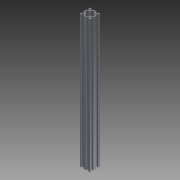
# Autodesk Inventor part: HFS5-4040-530
Saved by Autodesk Inventor 2015 (Build 190159000, 159)
## iProperties
Category: PARTsolutions
Company: MISUMI
Created: 2014-03-18
Part Number: HFS5-4040-530
Catalog Web Link: www.cadenas.de
Description: NFS5-4040, NFSB5-4040, HFS5-4040, HFSB5-4040, CAF5-4040, NFSF5-4040, HFSF5-4040,  HFST5-4040-HFS5 Series Aluminum Extrusions 40mm Square -2 Slots-
Vendor: MISUMI
Document SubType Name: Modeling
Designer: PARTuser1
Manufacturer: MISUMI
Density: 1 g/cm^3
Material: Generic
Appearance: RGB(175.94999939203154,175.94999939203154,175.94999939203154)
PSOL_IDENT_0: {\\10.0.0.236\data_v8\23d-libs\misumi\metric\38_al_extrusions_blackets\5\hfs5_4040.prj},542 {VTYP=3D
PSOL_IDENT_1: },{NB=HFS5-4040-530},{LINA=HFS5-4040-530},{NN=NFS5-4040, NFSB5-4040, HFS5-4040, HFSB5-4040, CAF5-404
PSOL_IDENT_2: 0, NFSF5-4040, HFSF5-4040,  HFST5-4040},{DATE=26.12.2013 07:39:21},{GEOMDATE=11.12.2013 08:22:00},{V
PSOL_IDENT_3: ERSION=},{LINEID=130},{LINESUBID=-1},{WBVAR=L,ALT1,ALT2,ALT4,ALT5,CP5,DL5,DR5,ALT6,HP6,NHL6,DL6,NHR6
PSOL_IDENT_4: ,DR6,ALT7,ALT8,ALT9,ALT10,ALT11,NH9,AH,BH,CH,DH,EH,NH10,AV,BV,CV,DV,EV,NH11,AP,BP,CP,DP,EP,ALT12,ALT
PSOL_IDENT_5: 13,Z,NH12,XA,XB,XC,XD,XE,NH13,YA,YB,YC,YD,YE,ALT16,HP16,DL16,DR16,ALT17,HQ17,JLP,ALT18,HQ18,KLP,ALT2
PSOL_IDENT_6: 0,ALT21,CHARSELECT1,CHARSELECT2}  {NB=HFS5-4040-530},{LINA=HFS5-4040-530},{KT=DUMMY},{PN=HFS5-4040-5
PSOL_IDENT_7: 30},{TPS=HFS5-4040},{MAT=A6N01SS-T5 Aluminum Alloy},{ST=Clear Anodize},{FRMW=40},{FRMH=40},{FRD=4.2}
PSOL_IDENT_8: ,{L=530.0},{MASS=1.28},{SA=472},{LX=8.89x10^4},{LY=8.89x10^4},{ALT1=},{M1=0},{DPL1=0},{DPR1=0},{ALT1
PSOL_IDENT_9: PN=},{ALT2=},{ALT2ALG= '','w/o End Tapping (Heli-Coil Insert)','LHP','with LHP (Tapping on the Left
PSOL_IDENT_10: (Heli-Coil Insert))','RHP','with RHP (Tapping on the Right (Heli-Coil Insert))','HPW','with HPW (Tap
PSOL_IDENT_11: ping on Both Ends (Heli-Coil Insert))' },{M2=0},{DP2=0},{ALT2PN=},{ALT4=},{ALT4ALG= '', 'w/o SC (Hig
PSOL_IDENT_12: h Precision Cut)', 'SC', 'with SC (High Precision Cut)' },{ALT4PN=},{ALT5=},{ALT5ALG= '','w/o 45 Deg
PSOL_IDENT_13: ree Cut','1','with 45 Degree Cut' },{CP5=},{CP5ALG= '','N/A' },{DL5=},{DL5ALG= '','N/A' },{DR5=},{DR
PSOL_IDENT_14: 5ALG= '','N/A' },{FRMALT5=0},{ALT5PN=},{ALT6=},{ALT6ALG= '','w/o Fastening Location Wrench Access Ho
PSOL_IDENT_15: le Alterations','1','with Fastening Location Wrench Access Hole Alterations' },{DD6=0.00},{HP6=},{HP
PSOL_IDENT_16: 6ALG= '','N/A' },{NHL6=},{NHL6ALG= '','N/A' },{DL6=},{DL6ALG= '','N/A' },{NHR6=},{NHR6ALG= '','N/A'
PSOL_IDENT_17: },{DR6=},{DR6ALG= '','N/A' },{HL6=0},{HR6=0},{J6=0},{K6=0},{ALT7=},{ALT7ALG= '','N/A' },{ALT8=},{ALT
PSOL_IDENT_18: 8ALG= '','N/A' },{ALT678PN=},{ALT9=},{ALT9ALG= '','w/o Location Specified Wrench Access Hole Alterat
PSOL_IDENT_19: ons (Horizontal)','1','with Location Specified Wrench Access Hole Alteratons (Horizontal)' },{ALT10=
PSOL_IDENT_20: },{ALT10ALG= '','w/o Location Specified Wrench Access Hole Alteratons (Vertical)','1','with Location
PSOL_IDENT_21: Specified Wrench Access Hole Alteratons (Vertical)' },{ALT11=},{ALT11ALG= '','w/o Location Specifie
PSOL_IDENT_22: d Wrench Access Hole Alteratons (Crisscross)','1','with Location Specified Wrench Access Hole Altera
PSOL_IDENT_23: tons (Crisscross)' },{DD9=0.00},{NH9=0},{NH9MAX=5},{NH9ALG=[0]},{AH=0.0},{AHMIN=7},{AHMAX=525},{AHAL
PSOL_IDENT_24: G=[0]},{BH=0.0},{BHMIN=2},{BHMAX=527},{BHALG=[0]},{CH=0.0},{CHMIN=2},{CHMAX=529},{CHALG=[0]},{DH=0.0
PSOL_IDENT_25: },{DHMIN=2},{DHMAX=531},{DHALG=[0]},{EH=0.0},{EHMIN=2},{EHMAX=523},{EHALG=[0]},{NH10=0},{NH10MAX=5},
PSOL_IDENT_26: {NH10ALG=[0]},{AV=0.0},{AVMIN=7},{AVMAX=525},{AVALG=[0]},{BV=0.0},{BVMIN=2},{BVMAX=527},{BVALG=[0]},
PSOL_IDENT_27: {CV=0.0},{CVMIN=2},{CVMAX=529},{CVALG=[0]},{DV=0.0},{DVMIN=2},{DVMAX=531},{DVALG=[0]},{EV=0.0},{EVMI
PSOL_IDENT_28: N=2},{EVMAX=523},{EVALG=[0]},{NH11=0},{NH11MAX=5},{NH11ALG=[0]},{AP=0.0},{APMIN=7},{APMAX=525},{APAL
PSOL_IDENT_29: G=[0]},{BP=0.0},{BPMIN=2},{BPMAX=527},{BPALG=[0]},{CP=0.0},{CPMIN=2},{CPMAX=529},{CPALG=[0]},{DP=0.0
PSOL_IDENT_30: },{DPMIN=2},{DPMAX=531},{DPALG=[0]},{EP=0.0},{EPMIN=2},{EPMAX=523},{EPALG=[0]},{ALT9PN=},{ALT10PN=},
PSOL_IDENT_31: {ALT11PN=},{ALT91011PN=},{ALT12=},{ALT12ALG= '','w/o Counterbore Hole in Specified Position (Vertica
PSOL_IDENT_32: l)','1','with Counterbore Hole in Specified Position (Vertical)' },{ALT13=},{ALT13ALG= '','w/o Count
PSOL_IDENT_33: erbore Hole in Specified Position (Horizontal)','1','with Counterbore Hole in Specified Position (Ho
PSOL_IDENT_34: rizontal)' },{Z=},{ZALG= '','N/A' },{DD12=0.0},{DD112=0.0},{NH12=0},{NH12MAX=5},{NH12ALG=[0]},{XA=0.
PSOL_IDENT_35: 0},{XAMIN=7},{XAMAX=525},{XAALG=[0]},{XB=0.0},{XBMIN=2},{XBMAX=527},{XBALG=[0]},{XC=0.0},{XCMIN=2},{
PSOL_IDENT_36: XCMAX=529},{XCALG=[0]},{XD=0.0},{XDMIN=2},{XDMAX=531},{XDALG=[0]},{XE=0.0},{XEMIN=2},{XEMAX=523},{XE
PSOL_IDENT_37: ALG=[0]},{NH13=0},{NH13MAX=5},{NH13ALG=[0]},{YA=0.0},{YAMIN=7},{YAMAX=525},{YAALG=[0]},{YB=0.0},{YBM
PSOL_IDENT_38: IN=2},{YBMAX=527},{YBALG=[0]},{YC=0.0},{YCMIN=2},{YCMAX=529},{YCALG=[0]},{YD=0.0},{YDMIN=2},{YDMAX=5
PSOL_IDENT_39: 31},{YDALG=[0]},{YE=0.0},{YEMIN=2},{YEMAX=523},{YEALG=[0]},{ALT12PN=},{ALT13PN=},{ALT1213PN=},{ALT16
PSOL_IDENT_40: =},{ALT16ALG= '','w/o M Type Hole Alteration','1','with M Type Hole Alteration' },{HP16=},{HP16ALG=
PSOL_IDENT_41: '','N/A' },{DL16=},{DL16ALG= '','N/A' },{DR16=},{DR16ALG= '','N/A' },{H116=0},{D16=0.0},{ALT16PN=},{
PSOL_IDENT_42: ALT17=},{ALT17ALG= '','w/o L Type Hole Alteration (Top)','1','with L Type Hole Alteration (Top)' },{
PSOL_IDENT_43: HQ17=0},{HQ17ALG=0},{JLP=0},{JLPMIN=4.9},{JLPMAX=0},{JLPALG=[0]},{L17=0},{D17=0.0},{ALT17PN=},{ALT18
PSOL_IDENT_44: =},{ALT18ALG= '','w/o L Type Hole Alteration (Bottom)','1','with L Type Hole Alteration (Bottom)' },
PSOL_IDENT_45: {HQ18=0},{HQ18ALG=0},{KLP=0},{KLPMIN=4.9},{KLPMAX=0},{KLPALG=[0]},{L18=0},{D18=0.0},{ALT18PN=},{ALT2
PSOL_IDENT_46: 0=},{ALT20PN=},{ALT21=},{CHARSELECT1=},{CS1=},{CHARSELECT2=},{CS2=},{ALT21PN=},{ERRORALT01=OK},{ERRO
PSOL_IDENT_47: RALT02=OK},{ERRORALT05=OK},{ERRORALT06091=OK},{ERRORALT06092=OK},{ERRORALT06093=OK},{ERRORALT06101=O
PSOL_IDENT_48: K},{ERRORALT06102=OK},{ERRORALT06103=OK},{ERRORALT06111=OK},{ERRORALT06112=OK},{ERRORALT06113=OK},{E
PSOL_IDENT_49: RRORALT06121=OK},{ERRORALT06122=OK},{ERRORALT06123=OK},{ERRORALT06131=OK},{ERRORALT06132=OK},{ERRORA
PSOL_IDENT_50: LT06133=OK},{ERRORALT0616=OK},{ERRORALT06171=OK},{ERRORALT06172=OK},{ERRORALT06173=OK},{ERRORALT0618
PSOL_IDENT_51: 1=OK},{ERRORALT06182=OK},{ERRORALT06183=OK},{ERRORALT0911=OK},{ERRORALT0913=OK},{ERRORALT0916=OK},{E
PSOL_IDENT_52: RRORALT0917=OK},{ERRORALT0918=OK},{ERRORALT1011=OK},{ERRORALT1012=OK},{ERRORALT1016=OK},{ERRORALT101
PSOL_IDENT_53: 7=OK},{ERRORALT1018=OK},{ERRORALT1112=OK},{ERRORALT1113=OK},{ERRORALT1116=OK},{ERRORALT1117=OK},{ERR
PSOL_IDENT_54: ORALT1118=OK},{ERRORALT1216=OK},{ERRORALT1217=OK},{ERRORALT1218=OK},{ERRORALT1316=OK},{ERRORALT1317=
PSOL_IDENT_55: OK},{ERRORALT1318=OK},{ERRORALT1617=OK},{ERRORALT1618=OK},{ERRORPN=}
SUPPLIER: MISUMI
ARTICLENO: HFS5-4040-530
BOMINFO: HFS5-4040-530
CREATOR: CADENAS GmbH
Title: HFS5-4040-530
Author: Cadenas PARTsolutions
Comments: HFS5 Series Aluminum Extrusions 40mm Square -2 Slots-
Autodesk Inventor part; units mm, degrees
sketch "Sketch_1" plane through (0, 0, 0) normal (0, 0, 1) x (1, 0, 0)
  arc A0 (-20, 13.3) -> (-19.7, 13) centre (-19.7, 13.3) ccw
  line L0 (-19.7, 13) -> (-18, 13)
  line L1 (-18, 13) -> (-18, 16)
  line L2 (-18, 16) -> (-17.0607, 16)
  line L3 (-17.0607, 16) -> (-14, 12.9393)
  line L4 (-14, 12.9393) -> (-14, 10.5196)
  line L5 (-14, 10.5196) -> (-13.7, 10)
  line L6 (-13.7, 10) -> (-14, 9.4804)
  line L7 (-14, 9.4804) -> (-14, 7.0607)
  line L8 (-14, 7.0607) -> (-17.0607, 4)
  line L9 (-17.0607, 4) -> (-18, 4)
  line L10 (-18, 4) -> (-18, 7)
  line L11 (-18, 7) -> (-19.7, 7)
  arc A1 (-19.7, 7) -> (-20, 6.7) centre (-19.7, 6.7) ccw
  line L12 (-20, 6.7) -> (-20, -6.7)
  arc A2 (-20, -6.7) -> (-19.7, -7) centre (-19.7, -6.7) ccw
  line L13 (-19.7, -7) -> (-18, -7)
  line L14 (-18, -7) -> (-18, -4)
  line L15 (-18, -4) -> (-17.0607, -4)
  line L16 (-17.0607, -4) -> (-14, -7.0607)
  line L17 (-14, -7.0607) -> (-14, -9.4804)
  line L18 (-14, -9.4804) -> (-13.7, -10)
  line L19 (-13.7, -10) -> (-14, -10.5196)
  line L20 (-14, -10.5196) -> (-14, -12.9393)
  line L21 (-14, -12.9393) -> (-17.0607, -16)
  line L22 (-17.0607, -16) -> (-18, -16)
  line L23 (-18, -16) -> (-18, -13)
  line L24 (-18, -13) -> (-19.7, -13)
  arc A3 (-19.7, -13) -> (-20, -13.3) centre (-19.7, -13.3) ccw
  line L25 (-20, -13.3) -> (-20, -19)
  arc A4 (-20, -19) -> (-19, -20) centre (-19, -19) ccw
  line L26 (-19, -20) -> (-13.3, -20)
  arc A5 (-13.3, -20) -> (-13, -19.7) centre (-13.3, -19.7) ccw
  line L27 (-13, -19.7) -> (-13, -18)
  line L28 (-13, -18) -> (-16, -18)
  line L29 (-16, -18) -> (-16, -17.0607)
  line L30 (-16, -17.0607) -> (-12.9393, -14)
  line L31 (-12.9393, -14) -> (-10.5196, -14)
  line L32 (-10.5196, -14) -> (-10, -13.7)
  line L33 (-10, -13.7) -> (-9.4804, -14)
  line L34 (-9.4804, -14) -> (-7.0607, -14)
  line L35 (-7.0607, -14) -> (-4, -17.0607)
  line L36 (-4, -17.0607) -> (-4, -18)
  line L37 (-4, -18) -> (-7, -18)
  line L38 (-7, -18) -> (-7, -19.7)
  arc A6 (-7, -19.7) -> (-6.7, -20) centre (-6.7, -19.7) ccw
  line L39 (-6.7, -20) -> (6.7, -20)
  arc A7 (6.7, -20) -> (7, -19.7) centre (6.7, -19.7) ccw
  line L40 (7, -19.7) -> (7, -18)
  line L41 (7, -18) -> (4, -18)
  line L42 (4, -18) -> (4, -17.0607)
  line L43 (4, -17.0607) -> (7.0607, -14)
  line L44 (7.0607, -14) -> (9.4804, -14)
  line L45 (9.4804, -14) -> (10, -13.7)
  line L46 (10, -13.7) -> (10.5196, -14)
  line L47 (10.5196, -14) -> (12.9393, -14)
  line L48 (12.9393, -14) -> (16, -17.0607)
  line L49 (16, -17.0607) -> (16, -18)
  line L50 (16, -18) -> (13, -18)
  line L51 (13, -18) -> (13, -19.7)
  arc A8 (13, -19.7) -> (13.3, -20) centre (13.3, -19.7) ccw
  line L52 (13.3, -20) -> (19, -20)
  arc A9 (19, -20) -> (20, -19) centre (19, -19) ccw
  line L53 (20, -19) -> (20, -13.3)
  arc A10 (20, -13.3) -> (19.7, -13) centre (19.7, -13.3) ccw
  line L54 (19.7, -13) -> (18, -13)
  line L55 (18, -13) -> (18, -16)
  line L56 (18, -16) -> (17.0607, -16)
  line L57 (17.0607, -16) -> (14, -12.9393)
  line L58 (14, -12.9393) -> (14, -10.5196)
  line L59 (14, -10.5196) -> (13.7, -10)
  line L60 (13.7, -10) -> (14, -9.4804)
  line L61 (14, -9.4804) -> (14, -7.0607)
  line L62 (14, -7.0607) -> (17.0607, -4)
  line L63 (17.0607, -4) -> (18, -4)
  line L64 (18, -4) -> (18, -7)
  line L65 (18, -7) -> (19.7, -7)
  arc A11 (19.7, -7) -> (20, -6.7) centre (19.7, -6.7) ccw
  line L66 (20, -6.7) -> (20, 6.7)
  arc A12 (20, 6.7) -> (19.7, 7) centre (19.7, 6.7) ccw
  line L67 (19.7, 7) -> (18, 7)
  line L68 (18, 7) -> (18, 4)
  line L69 (18, 4) -> (17.0607, 4)
  line L70 (17.0607, 4) -> (14, 7.0607)
  line L71 (14, 7.0607) -> (14, 9.4804)
  line L72 (14, 9.4804) -> (13.7, 10)
  line L73 (13.7, 10) -> (14, 10.5196)
  line L74 (14, 10.5196) -> (14, 12.9393)
  line L75 (14, 12.9393) -> (17.0607, 16)
  line L76 (17.0607, 16) -> (18, 16)
  line L77 (18, 16) -> (18, 13)
  line L78 (18, 13) -> (19.7, 13)
  arc A13 (19.7, 13) -> (20, 13.3) centre (19.7, 13.3) ccw
  line L79 (20, 13.3) -> (20, 19)
  arc A14 (20, 19) -> (19, 20) centre (19, 19) ccw
  line L80 (19, 20) -> (13.3, 20)
  arc A15 (13.3, 20) -> (13, 19.7) centre (13.3, 19.7) ccw
  line L81 (13, 19.7) -> (13, 18)
  line L82 (13, 18) -> (16, 18)
  line L83 (16, 18) -> (16, 17.0607)
  line L84 (16, 17.0607) -> (12.9393, 14)
  line L85 (12.9393, 14) -> (10.5196, 14)
  line L86 (10.5196, 14) -> (10, 13.7)
  line L87 (10, 13.7) -> (9.4804, 14)
  line L88 (9.4804, 14) -> (7.0607, 14)
  line L89 (7.0607, 14) -> (4, 17.0607)
  line L90 (4, 17.0607) -> (4, 18)
  line L91 (4, 18) -> (7, 18)
  line L92 (7, 18) -> (7, 19.7)
  arc A16 (7, 19.7) -> (6.7, 20) centre (6.7, 19.7) ccw
  line L93 (6.7, 20) -> (-6.7, 20)
  arc A17 (-6.7, 20) -> (-7, 19.7) centre (-6.7, 19.7) ccw
  line L94 (-7, 19.7) -> (-7, 18)
  line L95 (-7, 18) -> (-4, 18)
  line L96 (-4, 18) -> (-4, 17.0607)
  line L97 (-4, 17.0607) -> (-7.0607, 14)
  line L98 (-7.0607, 14) -> (-9.4804, 14)
  line L99 (-9.4804, 14) -> (-10, 13.7)
  line L100 (-10, 13.7) -> (-10.5196, 14)
  line L101 (-10.5196, 14) -> (-12.9393, 14)
  line L102 (-12.9393, 14) -> (-16, 17.0607)
  line L103 (-16, 17.0607) -> (-16, 18)
  line L104 (-16, 18) -> (-13, 18)
  line L105 (-13, 18) -> (-13, 19.7)
  arc A18 (-13, 19.7) -> (-13.3, 20) centre (-13.3, 19.7) ccw
  line L106 (-13.3, 20) -> (-19, 20)
  arc A19 (-19, 20) -> (-20, 19) centre (-19, 19) ccw
  line L107 (-20, 19) -> (-20, 13.3)
  line L108 (-18, 2) -> (-18, -2)
  line L109 (-18, -2) -> (-16.9393, -2)
  line L110 (-16.9393, -2) -> (-12.9393, -6)
  line L111 (-12.9393, -6) -> (-8.6694, -6)
  line L112 (-8.6694, -6) -> (-9.3371, -8.0074)
  arc A20 (-9.3371, -8.0074) -> (-8.0074, -9.3371) centre (-10, -10) ccw
  line L113 (-8.0074, -9.3371) -> (-6, -8.6694)
  line L114 (-6, -8.6694) -> (-6, -12.9393)
  line L115 (-6, -12.9393) -> (-2, -16.9393)
  line L116 (-2, -16.9393) -> (-2, -18)
  line L117 (-2, -18) -> (2, -18)
  line L118 (2, -18) -> (2, -16.9393)
  line L119 (2, -16.9393) -> (6, -12.9393)
  line L120 (6, -12.9393) -> (6, -8.6694)
  line L121 (6, -8.6694) -> (8.0074, -9.3371)
  arc A21 (8.0074, -9.3371) -> (9.3371, -8.0074) centre (10, -10) ccw
  line L122 (9.3371, -8.0074) -> (8.6694, -6)
  line L123 (8.6694, -6) -> (12.9393, -6)
  line L124 (12.9393, -6) -> (16.9393, -2)
  line L125 (16.9393, -2) -> (18, -2)
  line L126 (18, -2) -> (18, 2)
  line L127 (18, 2) -> (16.9393, 2)
  line L128 (16.9393, 2) -> (12.9393, 6)
  line L129 (12.9393, 6) -> (8.6694, 6)
  line L130 (8.6694, 6) -> (9.3371, 8.0074)
  arc A22 (9.3371, 8.0074) -> (8.0074, 9.3371) centre (10, 10) ccw
  line L131 (8.0074, 9.3371) -> (6, 8.6694)
  line L132 (6, 8.6694) -> (6, 12.9393)
  line L133 (6, 12.9393) -> (2, 16.9393)
  line L134 (2, 16.9393) -> (2, 18)
  line L135 (2, 18) -> (-2, 18)
  line L136 (-2, 18) -> (-2, 16.9393)
  line L137 (-2, 16.9393) -> (-6, 12.9393)
  line L138 (-6, 12.9393) -> (-6, 8.6694)
  line L139 (-6, 8.6694) -> (-8.0074, 9.3371)
  arc A23 (-8.0074, 9.3371) -> (-9.3371, 8.0074) centre (-10, 10) ccw
  line L140 (-9.3371, 8.0074) -> (-8.6694, 6)
  line L141 (-8.6694, 6) -> (-12.9393, 6)
  line L142 (-12.9393, 6) -> (-16.9393, 2)
  line L143 (-16.9393, 2) -> (-18, 2)
  constraints: 288 end point, 48 point on circle, 24 centre point
extrude "Extrusion1" add sketch "Sketch_1" against normal blind 530
ref_plane "to_frame_cap1_XY" through (0, 0, 0) normal (0, 0, 1) x (1, 0, 0)
ref_plane "to_frame_cap1_YZ" through (0, 0, 0) normal (1, 0, 0) x (0, 1, 0)
ref_plane "to_frame_cap1_ZX" through (0, 0, 0) normal (0, 1, 0) x (0, 0, 1)
ref_plane "C1_XY" through (0, 0, 0) normal (0, 0, 1) x (1, 0, 0)
ref_plane "C1_YZ" through (0, 0, 0) normal (1, 0, 0) x (0, 1, 0)
ref_plane "C1_ZX" through (0, 0, 0) normal (0, 1, 0) x (0, 0, 1)
ref_plane "to_frame_cap2_XY" through (0, 0, -530) normal (0, 0, -1) x (1, 0, 0)
ref_plane "to_frame_cap2_YZ" through (0, 0, -530) normal (1, 0, 0) x (0, -1, 0)
ref_plane "to_frame_cap2_ZX" through (0, 0, -530) normal (0, -1, 0) x (0, 0, -1)
body "Solid1"
